AIoTNode (Autodesk Fusion 360 archive; units mm, degrees)
design "FRAME-BMS"
part number: 2026-03-19-13-46-00-804
Autodesk Fusion 360 part; units mm, degrees
sketch "Sketch1" plane through (0, 0, 0) normal (1, 0, 0) x (0, 1, 0)
  line L0 (10, 72) -> (70, 72)
  line L1 (70, 72) -> (70, 5)
  line L2 (70, 5) -> (10, 5)
  line L3 (10, 5) -> (10, 72)
  dimension "d1" = 10
  dimension "d2" = 5
  dimension "d3" = 60
  dimension "d4" = 67
  constraint horizontal L0
  constraint vertical L1
  constraint horizontal L2
  constraint vertical L3
  measures "d1" horizontal distance of origin L2.end
  measures "d2" vertical distance of origin L2.end
  measures "d3" distance of L1.end L2.end
  measures "d4" distance of L0.start L2.end
extrude "Extrude1" add sketch "Sketch1" along normal blind 2 makes body 1
sketch "Sketch2" plane through (2, 0, 0) normal (1, 0, 0) x (0, 1, 0)
  line L0 (10, 5) -> (70, 5)
  line L1 (70, 5) -> (70, 72)
  line L2 (70, 72) -> (10, 72)
  line L3 (10, 72) -> (10, 5)
  circle A0 centre (16.5, 11.5) radius 4.5
  dimension "d7" = 9
  dimension "d8" = 6.5
  dimension "d9" = 6.5
  measures "d7" diameter of A0
  measures "d8" horizontal distance of L0.start A0.centre
  measures "d9" vertical distance of L0.start A0.centre
extrude "Extrude2" add sketch "Sketch2" along normal blind 4 draft -15 separate body contours A0 makes body 2
hole "Hole1" at (6, 16.5, 11.5) direction (-1, 0, 0) diameter 3.85 depth 4.5 tip angle 180 bodies 2
pattern_linear "R-Pattern1" count 2 spacing 54 along (0, 0, 1) count 2 spacing 47 along (0, 1, 0) of bodies 2 makes body 3 at (2.8889, 12.2382, 65.5) makes body 4 at (2.8889, 63.1815, 7.2501) makes body 5 at (2.8889, 59.2382, 65.5)
sketch "Sketch3" plane through (0, 0, 0) normal (-1, 0, 0) x (0, -1, 0)
  line L0 (-70, 5) -> (-10, 5)
  line L1 (-10, 5) -> (-10, 72)
  line L2 (-10, 72) -> (-70, 72)
  line L3 (-70, 72) -> (-70, 5)
  line L4 (-70, 5) -> (-58, 5)
  line L5 (-58, 5) -> (-58, 8)
  line L6 (-58, 8) -> (-70, 8)
  line L7 (-70, 8) -> (-70, 5)
  constraint horizontal L4
  constraint vertical L5
  constraint horizontal L6
  constraint vertical L7
  constraint coincident L0.start L3.end
extrude "Extrude3" add sketch "Sketch3" along normal blind 8 separate body contours L0 L3 L4 L5 L6 L7 makes body 6
sketch "Sketch4" plane through (0, 0, 0) normal (0, 1, 0) x (1, 0, 0)
  line L0 (-6, -8) -> (0, -8)
  line L1 (0, -8) -> (0, -14)
  line L2 (0, -14) -> (-6, -8)
  constraint horizontal L0
  constraint perpendicular L0 L1
extrude "Extrude4" add sketch "Sketch4" along normal blind 2 separate body makes body 7
move_body "Move3" bodies 7 to x (1, 0, 0) y (0, 1, 0) z (0, 0, 1) at (0, 68, 0)
copy_body "CopyPasteBodies3" bodies 7 makes body 8
move_body "Move4" bodies 8 to x (1, 0, 0) y (0, 1, 0) z (0, 0, 1) at (0, -10, 0)
hole "Hole2" at (-4, 64, 8) direction (0, 0, -1) diameter 3 depth 3 tip angle 180 counterbore diameter 4 counterbore depth 1.5 bodies 6
copy_body "CopyPasteBodies4" bodies 6 7 8 makes body 9 makes body 10 makes body 11
move_body "Move5" bodies 9 10 11 to x (1, 0, 0) y (0, 1, 0) z (0, 0, 1) at (0, -48, 0)
copy_body "CopyPasteBodies5" bodies 6 8 7 makes body 12 makes body 13 makes body 14
move_body "Move6" bodies 12 13 14 to x (1, 0, 0) y (0, 1, 0) z (0, 0, 1) at (0, -16, 0)
copy_body "CopyPasteBodies6" bodies 12 13 14 makes body 15 makes body 16 makes body 17
move_body "Move7" bodies 15 16 17 to x (1, 0, 0) y (0, 1, 0) z (0, 0, 1) at (0, -16, 0)
move_body "Move8" bodies 12 13 14 15 16 17 to x (1, 0, 0) y (0, 1, 0) z (0, 0, 1) at (0, 0, 58)
move_body "Move9" bodies 9 6 7 11 10 8 to x (1, 0, 0) y (0, 1, 0) z (0, 0, 1) at (0, 0, 12)
move_body "Move10" bodies 12 15 14 16 17 13 to x (1, 0, 0) y (0, 1, 0) z (0, 0, 1) at (0, 0, -12)
sketch "Sketch5" plane through (0, 0, 0) normal (-1, 0, 0) x (0, -1, 0)
  line L0 (-70, 5) -> (-10, 5)
  line L1 (-10, 5) -> (-10, 72)
  line L2 (-10, 72) -> (-70, 72)
  line L3 (-70, 72) -> (-70, 5)
  line L4 (-70, 60) -> (-67, 57)
  line L5 (-67, 57) -> (-67, 30)
  line L6 (-67, 30) -> (-70, 27)
  line L7 (-70, 27) -> (-70, 60)
  line L8 (-10, 27) -> (-10, 60)
  line L9 (-13, 30) -> (-10, 27)
  line L10 (-13, 57) -> (-13, 30)
  line L11 (-10, 60) -> (-13, 57)
  dimension "d34" = 33
  dimension "d35" = 12
  dimension "d36" = 33
  dimension "d37" = 12
  dimension "d38" = 3
  dimension "d39" = 3
  constraint coincident L3 L4.start
  constraint parallel L3 L5
  constraint coincident L3 L6.end
  constraint perpendicular L4 L6
  measures "d34" distance of L4.start L6.end
  measures "d35" distance of L2.end L4.start
  measures "d36" distance of L8.end L8.start
  measures "d37" distance of L1.end L8.end
  measures "d38" distance of L5 L7
  measures "d39" distance of L8 L10
extrude "Extrude5" cut sketch "Sketch5" against normal up to surface (2 mm away) contours L3 L4 L5 L6 L7 | L1 L8 L9 L10 L11 bodies 1

design "Magnet"
part number: 2026-03-19-21-53-07-206
Autodesk Fusion 360 part; units mm, degrees
sketch "Sketch1" plane through (0, 0, 0) normal (0, 0, 1) x (1, 0, 0)
  circle A0 centre (0, 0) radius 8
  dimension "d1" = 16
  constraint coincident A0.centre origin
  measures "d1" diameter of A0
extrude "Extrude1" add sketch "Sketch1" along normal blind 4.5
sketch "Sketch2" plane through (0, 0, 4.5) normal (0, 0, 1) x (-1, 0, 0)
  circle A0 centre (0, 0) radius 8
  circle A1 centre (0, 0) radius 2
  dimension "d4" = 4
  constraint concentric A0 A1
  measures "d4" diameter of A1
extrude "Extrude2" add sketch "Sketch2" along normal blind 8 contours A1

design "Battery-Pack" references "Battery-Pack"
part number: 2026-03-20-16-38-44-080
Autodesk Fusion 360 part; units mm, degrees
sketch "Sketch1" plane through (0, 0, 0) normal (1, 0, 0) x (0, 1, 0)
  line L0 (-8.65, 0) -> (-46.65, 0)
  line L1 (-46.65, 18.7) -> (-8.65, 18.7)
  arc A0 (-8.65, 0) -> (-8.65, 18.7) centre (-8.65, 9.35) ccw
  arc A1 (-46.65, 18.7) -> (-46.65, 0) centre (-46.65, 9.35) ccw
  constraint horizontal L0
  constraint horizontal L1
extrude "Extrude1" add sketch "Sketch1" along normal blind 67

design "Swtich"
part number: 2026-03-20-21-33-23-195
Autodesk Fusion 360 part; units mm, degrees
sketch "Sketch1" plane through (0, 0, 0) normal (0, 0, 1) x (1, 0, 0)
  circle A0 centre (0, 0) radius 5
  dimension "d1" = 10
  constraint coincident A0.centre origin
  measures "d1" diameter of A0
extrude "Extrude1" add sketch "Sketch1" along normal blind 10
sketch "Sketch3" plane through (0, 0, 0) normal (0, 1, 0) x (1, 0, 0)
  arc A0 (0, -16.9) -> (4, -15.6223) centre (0, -10) ccw
  line L0 (0, -10) -> (6, -10)
  line L1 (0, -16.9) -> (0, -10)
  line L2 (6, -10) -> (6, -13.4073)
  line L3 (6, -13.4073) -> (6, -15.615)
  line L4 (6, -15.615) -> (4, -15.6223)
  constraint coincident A0.centre L0.start
  constraint horizontal L0
  constraint perpendicular L0 L1
  constraint perpendicular L0 L2
revolve "Revolve1" add sketch "Sketch3" angle 360 about axis through (0, 0, 16.9) along (0, 0, -1)
sketch "Sketch4" plane through (0, 0, 0) normal (0, 0, 1) x (1, 0, 0)
  line L0 (-1.15, 0.75) -> (-1.65, 0.75)
  line L1 (-1.15, -0.75) -> (-1.65, -0.75)
  line L2 (-1.15, 0.75) -> (-1.15, -0.75)
  line L3 (-1.65, 0.75) -> (-1.65, -0.75)
  line L4 (1.15, 0.75) -> (1.65, 0.75)
  line L5 (1.15, -0.75) -> (1.65, -0.75)
  line L6 (1.65, 0.75) -> (1.65, -0.75)
  line L7 (1.15, 0.75) -> (1.15, -0.75)
  constraint horizontal L0
  constraint perpendicular L0 L2
  constraint perpendicular L1 L3
extrude "Extrude2" add sketch "Sketch4" against normal blind 6

design "FRAME-BATTERY" references "FRAME-BATTERY"
part number: 2026-03-20-22-12-17-539
Autodesk Fusion 360 part; units mm, degrees
sketch "Sketch1" plane through (0, 0, 0) normal (0, 0, 1) x (1, 0, 0)
  line L0 (97.5, 72) -> (27.5, 72)
  line L1 (27.5, 72) -> (27.5, 3)
  line L2 (27.5, 3) -> (97.5, 3)
  line L3 (97.5, 72) -> (97.5, 3)
  dimension "d10" = 27.5
  dimension "d11" = 3
  dimension "d12" = 70
  dimension "d13" = 69
  constraint horizontal L0
  constraint vertical L1
  constraint horizontal L2
  constraint perpendicular L2 L3
  measures "d10" horizontal distance of origin L1.end
  measures "d11" vertical distance of origin L1.end
  measures "d12" distance of L0.start L0.end
  measures "d13" distance of L0.start L2.end
extrude "Extrude1" add sketch "Sketch1" along normal blind 3.5 makes body 1
hole "Hole1" at (32.5, 69, 3.5) direction (0, 0, -1) diameter 3 depth 3.5 tip angle 180 counterbore diameter 4 counterbore depth 2.5 bodies 1
pattern_linear "R-Pattern1" count 2 spacing 60 along (1, 0, 0) count 2 spacing 63 along (0, -1, 0) of "Hole1"
sketch "Sketch2" plane through (0, 0, 3.5) normal (0, 0, 1) x (-1, 0, 0)
  circle A0 centre (-92.5, -6) radius 2
  circle A1 centre (-32.5, -6) radius 2
  circle A2 centre (-92.5, -69) radius 2
  circle A3 centre (-32.5, -69) radius 2
  line L0 (-27.5, -72) -> (-27.5, -3)
  line L1 (-27.5, -3) -> (-97.5, -3)
  line L2 (-97.5, -3) -> (-97.5, -72)
  line L3 (-97.5, -72) -> (-27.5, -72)
  line L4 (-27.5, -72) -> (-97.5, -3)
  line L5 (-97.5, -72) -> (-27.5, -3)
  line L6 (-37, -69) -> (-37, -70)
  line L7 (-88, -69) -> (-88, -70)
  line L8 (-37, -70) -> (-88, -70)
  line L9 (-88, -69) -> (-37, -69)
  line L10 (-62.5, -37.5) -> (-97.5, -37.5)
  constraint coincident L0.start L3.end
  constraint coincident L1.end L2.start
  constraint coincident L2.end L3.start
  constraint coincident L0.end L1.start
  constraint vertical L6
  constraint vertical L7
  constraint perpendicular L7 L8
  constraint perpendicular L6 L9
  constraint midpoint L4 L10.start
  constraint midpoint L2 L10.end
extrude "Extrude2" add sketch "Sketch2" along normal blind 1 separate body contours L6 L7 L8 L9 makes body 2
ref_plane "WorkPlane1" through (0, 37.5, 0) normal (0, 1, 0) x (0, 0, 1)
mirror "Mirror1" about plane through (0, 37.5, 0) normal (0, 1, 0) of bodies 2 makes body 3

design "1rmb"
part number: 2026-03-20-23-18-56-402
Autodesk Fusion 360 part; units mm, degrees
sketch "Sketch1" plane through (0, 0, 0) normal (0, 1, 0) x (1, 0, 0)
  circle A0 centre (-39.3328, -19.6664) radius 11.125
  dimension "d1" = 22.25
  measures "d1" diameter of A0
extrude "Extrude1" add sketch "Sketch1" along normal blind 2.4 makes body 1
move_body "Move1" bodies 1 to x (1, 0, 0) y (0, 1, 0) z (0, 0, 1) at (-36, 0, -8)
sketch "Sketch2" plane through (0, 0, 0) normal (0, 0, 1) x (1, 0, 0)
  circle A0 centre (-80, 40) radius 11.125
  dimension "d4" = 22.25
  measures "d4" diameter of A0
extrude "Extrude2" add sketch "Sketch2" along normal blind 2.4 separate body makes body 2
move_body "Align1" bodies 1 to x (1, 0, 0) y (0, 1, 0) z (0, 0, 1) at (-4.6672, 38.8, 0)
move_face "MoveFace1" by (0, 0, 2.4) 1 faces at (-83.6669, 38.8, 7.1745) on bodies 1
move_body "Move2" bodies 1 to x (1, 0, 0) y (0, 1, 0) z (0, 0, 1) at (0, 0, 2.4)
move_body "Move3" bodies 1 to x (1, 0, 0) y (0, 1, 0) z (0, 0, 1) at (0, -1.2, 0)
